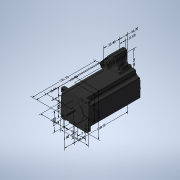
# Autodesk Inventor part: 8156180 EMMT-ST-57-L-RS---(400)
Saved by Autodesk Inventor 2021 (Build 250183000, 183)
## iProperties
Created: 2026-04-24
Part Number: 8156180 EMMT-ST-57-L-RS---(400)
Material: Generic
Catalog Web Link: www.3dfindit.com
Description: EMMT-ST-stepper motor
Vendor: FESTO
Document SubType Name: Modeling
Designer: psAdmin
Manufacturer: FESTO
Mass: 1260 g
Surface Area: 351.744 cm^2
Volume: 333.112 cm^3
Density: 1 g/cm^3
Appearance: PSOLRGB-176-176-176
Category: PARTsolutions
Company: FESTO
Title: 8156180 EMMT-ST-57-L-RS
Author: Cadenas PARTsolutions
Comments: stepper motor
PSOL_IDENT_0: {$CADENAS_DATA/23d-libs/festo/parts/e/emmt/emmt_st.prj},199 {VTYP=3D},{NB=8156180 EMMT-ST-57-L-RS---
PSOL_IDENT_1: (400)},{LINA=8156180 EMMT-ST-57-L-RS},{NN=EMMT-ST},{DATE=09.12.2025 15:36:59},{GEOMDATE=09.12.2025 1
PSOL_IDENT_2: 5:36:20},{VERSION=},{LINEID=200},{WBVAR=LOG},{WBNUMERIC=}  {NB=8156180 EMMT-ST-57-L-RS---(400)},{LIN
PSOL_IDENT_3: A=8156180 EMMT-ST-57-L-RS},{KT=DUMMY},{TNR=8156180},{TYP=EMMT-ST-57-L-RS},{FLA=57},{BAU=L},{ELE=R},{
PSOL_IDENT_4: BRE=-},{LOGDEST=mechanical},{LOG=400},{LOGX='400','High', '300', 'Medium', '200', 'Low'},{B1=56.400}
PSOL_IDENT_5: ,{B2=47.140},{D1=6.350},{D2=38.100},{D3=M17},{D3N=17.000},{D4=5},{D4N=5.000},{H1=88.000},{H3=49.300}
PSOL_IDENT_6: ,{L=131.100},{L1=110.500},{L2=20.600},{L3=1.600},{L4=5.000},{L5=16.700},{L6=33.400},{L7=11.000},{R=3
PSOL_IDENT_7: .000},{L8=0.000},{CNSMASSEXACT=1.260},{GTIN=4052568639686}
NB: 8156180 EMMT-ST-57-L-RS---(400)
NN: EMMT-ST
NT: stepper motor
NBSYN: $TNR. $TYP.---($LOG.)
LINA: 8156180 EMMT-ST-57-L-RS
CATALOG: Festo
TNR: 8156180
TYP: EMMT-ST-57-L-RS
LOG: High
B1: 56.4
B2: 47.14
D1: 6.35
D2: 38.1
D3: M17
D4: 5
H1: 88
H3: 49.3
L: 131.1
L1: 110.5
L2: 20.6
L3: 1.6
L4: 5
L5: 16.7
L6: 33.4
L7: 11
R: 3
CNSMASSEXACT: 1.26
GTIN: 4052568639686
SUPPLIER: FESTO
ARTICLENO: 8156180 EMMT-ST-57-L-RS---(400)
BOMINFO: 8156180 EMMT-ST-57-L-RS
CREATOR: CADENAS GmbH
Autodesk Inventor part; units mm, degrees
sketch "Sketch_1" plane through (0, 0, 0) normal (0, 0, 1) x (1, 0, 0)
  line L0 (-28.2, -28.2) -> (28.2, -28.2)
  line L1 (28.2, -28.2) -> (28.2, 28.2)
  line L2 (28.2, 28.2) -> (-28.2, 28.2)
  line L3 (-28.2, 28.2) -> (-28.2, -28.2)
  constraints: 8 end point
extrude "Extrusion1" add sketch "Sketch_1" against normal blind 110.5
sketch "Sketch_2" plane through (0, 0, -5) normal (0, 0, 1) x (1, 0, 0)
  line L0 (-33.2, -33.2) -> (33.2, -33.2)
  line L1 (33.2, -33.2) -> (33.2, 33.2)
  line L2 (33.2, 33.2) -> (-33.2, 33.2)
  line L3 (-33.2, 33.2) -> (-33.2, -33.2)
  line L4 (-28.2, 19) -> (-28.2, -19)
  line L5 (-28.2, -19) -> (-24, -19)
  arc A0 (-19, -24) -> (-24, -19) centre (-24, -24) ccw
  line L6 (-19, -24) -> (-19, -28.2)
  line L7 (-19, -28.2) -> (19, -28.2)
  line L8 (19, -28.2) -> (19, -24)
  arc A1 (24, -19) -> (19, -24) centre (24, -24) ccw
  line L9 (24, -19) -> (28.2, -19)
  line L10 (28.2, -19) -> (28.2, 19)
  line L11 (28.2, 19) -> (24, 19)
  arc A2 (19, 24) -> (24, 19) centre (24, 24) ccw
  line L12 (19, 24) -> (19, 28.2)
  line L13 (19, 28.2) -> (-19, 28.2)
  line L14 (-19, 28.2) -> (-19, 24)
  arc A3 (-24, 19) -> (-19, 24) centre (-24, 24) ccw
  line L15 (-24, 19) -> (-28.2, 19)
  constraints: 32 end point, 8 point on circle, 4 centre point
extrude "Extrusion2" cut sketch "Sketch_2" against normal blind 105.5
sketch "Sketch_3" plane through (0, 0, -5) normal (0, 0, 1) x (1, 0, 0)
  line L0 (-33.2, -33.2) -> (33.2, -33.2)
  line L1 (33.2, -33.2) -> (33.2, 33.2)
  line L2 (33.2, 33.2) -> (-33.2, 33.2)
  line L3 (-33.2, 33.2) -> (-33.2, -33.2)
  line L4 (-28.2, 16.8) -> (-28.2, -16.8)
  arc A0 (-28.2, -16.8) -> (-26, -19) centre (-26, -16.8) ccw
  line L5 (-26, -19) -> (-24, -19)
  arc A1 (-19, -24) -> (-24, -19) centre (-24, -24) ccw
  line L6 (-19, -24) -> (-19, -26)
  arc A2 (-19, -26) -> (-16.8, -28.2) centre (-16.8, -26) ccw
  line L7 (-16.8, -28.2) -> (16.8, -28.2)
  arc A3 (16.8, -28.2) -> (19, -26) centre (16.8, -26) ccw
  line L8 (19, -26) -> (19, -24)
  arc A4 (24, -19) -> (19, -24) centre (24, -24) ccw
  line L9 (24, -19) -> (26, -19)
  arc A5 (26, -19) -> (28.2, -16.8) centre (26, -16.8) ccw
  line L10 (28.2, -16.8) -> (28.2, 16.8)
  arc A6 (28.2, 16.8) -> (26, 19) centre (26, 16.8) ccw
  line L11 (26, 19) -> (24, 19)
  arc A7 (19, 24) -> (24, 19) centre (24, 24) ccw
  line L12 (19, 24) -> (19, 26)
  arc A8 (19, 26) -> (16.8, 28.2) centre (16.8, 26) ccw
  line L13 (16.8, 28.2) -> (-16.8, 28.2)
  arc A9 (-16.8, 28.2) -> (-19, 26) centre (-16.8, 26) ccw
  line L14 (-19, 26) -> (-19, 24)
  arc A10 (-24, 19) -> (-19, 24) centre (-24, 24) ccw
  line L15 (-24, 19) -> (-26, 19)
  arc A11 (-26, 19) -> (-28.2, 16.8) centre (-26, 16.8) ccw
  constraints: 32 end point, 24 point on circle, 12 centre point
extrude "Extrusion3" cut sketch "Sketch_3" against normal blind 105.5
sketch "Sketch_4" plane through (0, 0, 0) normal (0, 0, 1) x (1, 0, 0)
  line L0 (-33.2, -33.2) -> (33.2, -33.2)
  line L1 (33.2, -33.2) -> (33.2, 33.2)
  line L2 (33.2, 33.2) -> (-33.2, 33.2)
  line L3 (-33.2, 33.2) -> (-33.2, -33.2)
  line L4 (-28.2, 25.2) -> (-28.2, -25.2)
  arc A0 (-28.2, -25.2) -> (-25.2, -28.2) centre (-25.2, -25.2) ccw
  line L5 (-25.2, -28.2) -> (25.2, -28.2)
  arc A1 (25.2, -28.2) -> (28.2, -25.2) centre (25.2, -25.2) ccw
  line L6 (28.2, -25.2) -> (28.2, 25.2)
  arc A2 (28.2, 25.2) -> (25.2, 28.2) centre (25.2, 25.2) ccw
  line L7 (25.2, 28.2) -> (-25.2, 28.2)
  arc A3 (-25.2, 28.2) -> (-28.2, 25.2) centre (-25.2, 25.2) ccw
  constraints: 16 end point, 8 point on circle, 4 centre point
extrude "Extrusion4" cut sketch "Sketch_4" against normal blind 5
sketch "Sketch5" plane through (0, 0, 0) normal (0, 0, 1) x (1, 0, 0)
  point P0 (23.57, 23.57)
hole "Hole1" at (23.57, 23.57, 0) direction (0, 0, -1) diameter 5 depth 5 countersink diameter 6 countersink angle 90
sketch "Sketch6" plane through (0, 0, 0) normal (0, 0, 1) x (1, 0, 0)
  point P0 (23.57, -23.57)
hole "Hole2" at (23.57, -23.57, 0) direction (0, 0, -1) diameter 5 depth 5 countersink diameter 6 countersink angle 90
sketch "Sketch7" plane through (0, 0, 0) normal (0, 0, 1) x (1, 0, 0)
  point P0 (-23.57, 23.57)
hole "Hole3" at (-23.57, 23.57, 0) direction (0, 0, -1) diameter 5 depth 5 countersink diameter 6 countersink angle 90
sketch "Sketch8" plane through (0, 0, 0) normal (0, 0, 1) x (1, 0, 0)
  point P0 (-23.57, -23.57)
hole "Hole4" at (-23.57, -23.57, 0) direction (0, 0, -1) diameter 5 depth 5 countersink diameter 6 countersink angle 90
sketch "Sketch_9" plane through (0, 0, 0) normal (0, 0, 1) x (1, 0, 0)
  arc A0 (12.339, 25.045) -> (18.839, 25.045) centre (15.589, 25.045) ccw
  line L0 (18.839, 25.045) -> (18.839, 28.2)
  line L1 (18.839, 28.2) -> (12.339, 28.2)
  line L2 (12.339, 28.2) -> (12.339, 25.045)
  constraints: 6 end point, 2 point on circle, 1 centre point
extrude "Extrusion5" cut sketch "Sketch_9" against normal blind 2.5
sketch "Sketch_10" plane through (0, 0, 0) normal (0, 0, 1) x (1, 0, 0)
  line L0 (-28.2, 18.839) -> (-28.2, 12.339)
  line L1 (-28.2, 12.339) -> (-25.045, 12.339)
  arc A0 (-25.045, 12.339) -> (-25.045, 18.839) centre (-25.045, 15.589) ccw
  line L2 (-25.045, 18.839) -> (-28.2, 18.839)
  constraints: 6 end point, 2 point on circle, 1 centre point
extrude "Extrusion6" cut sketch "Sketch_10" against normal blind 2.5
sketch "Sketch_11" plane through (0, 0, 0) normal (0, 0, 1) x (1, 0, 0)
  line L0 (-18.839, -25.045) -> (-18.839, -28.2)
  line L1 (-18.839, -28.2) -> (-12.339, -28.2)
  line L2 (-12.339, -28.2) -> (-12.339, -25.045)
  arc A0 (-12.339, -25.045) -> (-18.839, -25.045) centre (-15.589, -25.045) ccw
  constraints: 6 end point, 2 point on circle, 1 centre point
extrude "Extrusion7" cut sketch "Sketch_11" against normal blind 2.5
sketch "Sketch_12" plane through (0, 0, 0) normal (0, 0, 1) x (1, 0, 0)
  arc A0 (25.045, -12.339) -> (25.045, -18.839) centre (25.045, -15.589) ccw
  line L0 (25.045, -18.839) -> (28.2, -18.839)
  line L1 (28.2, -18.839) -> (28.2, -12.339)
  line L2 (28.2, -12.339) -> (25.045, -12.339)
  constraints: 6 end point, 2 point on circle, 1 centre point
extrude "Extrusion8" cut sketch "Sketch_12" against normal blind 2.5
sketch "Sketch_13" plane through (15.589, 0, 0) normal (1, 0, 0) x (0, 0, -1)
  line L0 (2.5, 25.045) -> (0.5, 25.045)
  line L1 (0.5, 25.045) -> (0.5, 27.5284)
  arc A0 (0.5913, 27.628) -> (0.5, 27.5284) centre (0.6, 27.5284) ccw
  line L2 (0.5913, 27.628) -> (2.5, 27.795)
  line L3 (2.5, 27.795) -> (2.5, 25.045)
  line L4 (2.5, 25.045) -> (0.5, 25.045)
  constraints: 10 end point, 2 point on circle, 1 centre point
revolve "Revolution1" add sketch "Sketch_13" angle 360 about axis through (15.589, 25.045, -2.5) along (0, 0, -1)
pattern_linear "Rectangular Pattern1" count 2 spacing 41.7198 along (-0.9739751, -0.2266552, 0) count 2 spacing 41.7198 along (0.2266552, -0.9739751, 0) of "Revolution1"
sketch "Sketch_15" plane through (15.589, 25.045, -0.5) normal (0, 0, 1) x (0, 1, 0)
  line L0 (-2.75, -0.4) -> (2.75, -0.4)
  line L1 (2.75, -0.4) -> (2.75, 0.4)
  line L2 (2.75, 0.4) -> (-2.75, 0.4)
  line L3 (-2.75, 0.4) -> (-2.75, -0.4)
  constraints: 8 end point
extrude "Extrusion9" cut sketch "Sketch_15" against normal blind 0.85
sketch "Pattern_2_SKETCH_1" plane through (-25.045, 15.589, -0.5) normal (0, 0, 1) x (0, 1, 0)
  line L0 (-2.75, -0.4) -> (2.75, -0.4)
  line L1 (2.75, -0.4) -> (2.75, 0.4)
  line L2 (2.75, 0.4) -> (-2.75, 0.4)
  line L3 (-2.75, 0.4) -> (-2.75, -0.4)
  constraints: 8 end point
sketch "Pattern_2_SKETCH_2" plane through (-25.045, 15.589, -0.5) normal (0, 0, 1) x (0, 1, 0)
  line L0 (-43.383, -9.856) -> (-37.883, -9.856)
  line L1 (-37.883, -9.856) -> (-37.883, -9.056)
  line L2 (-37.883, -9.056) -> (-43.383, -9.056)
  line L3 (-43.383, -9.056) -> (-43.383, -9.856)
  constraints: 8 end point
sketch "Pattern_2_SKETCH_3" plane through (-25.045, 15.589, -0.5) normal (0, 0, 1) x (0, 1, 0)
  line L0 (-33.928, -50.49) -> (-28.428, -50.49)
  line L1 (-28.428, -50.49) -> (-28.428, -49.69)
  line L2 (-28.428, -49.69) -> (-33.928, -49.69)
  line L3 (-33.928, -49.69) -> (-33.928, -50.49)
  constraints: 8 end point
extrude "Extrusion10" cut sketch "Pattern_2_SKETCH_1" against normal blind 0.85
extrude "Extrusion11" cut sketch "Pattern_2_SKETCH_2" against normal blind 0.85
extrude "Extrusion12" cut sketch "Pattern_2_SKETCH_3" against normal blind 0.85
sketch "Sketch_17" plane through (0, 0, 0) normal (1, 0, 0) x (0, 1, 0)
  line L0 (0, 0) -> (0, 1.6)
  line L1 (0, 1.6) -> (18.8, 1.6)
  line L2 (18.8, 1.6) -> (19.05, 1.35)
  line L3 (19.05, 1.35) -> (19.05, 0)
  line L4 (19.05, 0) -> (0, 0)
  line L5 (0, 0) -> (0, 1.6)
  constraints: 12 end point
revolve "Revolution2" add sketch "Sketch_17" angle 360 about axis through (0, 0, 0) along (0, 0, -1)
sketch "Sketch19" plane through (0, 0, 1.6) normal (0, 0, 1) x (1, 0, 0)
  point P0 (0, 0)
hole "Hole5" at (0, 0, 1.6) direction (0, 0, -1) diameter 9 depth 5 countersink diameter 10 countersink angle 90
sketch "Sketch_19" plane through (0, 0, 0) normal (1, 0, 0) x (0, 1, 0)
  line L0 (0, -5.4) -> (0, 18.8783)
  line L1 (0, 18.8783) -> (1.25, 19.6)
  line L2 (1.25, 19.6) -> (1.25, 20.6)
  line L3 (1.25, 20.6) -> (2.875, 20.6)
  line L4 (2.875, 20.6) -> (3.175, 20.3)
  line L5 (3.175, 20.3) -> (3.175, -1.4)
  arc A0 (3.175, -1.4) -> (5.175, -3.4) centre (5.175, -1.4) ccw
  line L6 (5.175, -3.4) -> (5.175, -5.4)
  line L7 (5.175, -5.4) -> (0, -5.4)
  line L8 (0, -5.4) -> (0, 18.8783)
  constraints: 18 end point, 2 point on circle, 1 centre point
revolve "Revolution3" add sketch "Sketch_19" angle 360 about axis through (0, 0, -5.4) along (0, 0, -1)
sketch "Sketch_20" plane through (0, 0, 0) normal (1, 0, 0) x (0, 1, 0)
  line L0 (0, -115.5) -> (0, -110.5)
  line L1 (0, -110.5) -> (19.5, -110.5)
  arc A0 (19.5, -110.5) -> (19.9094, -110.287) centre (19.5, -110) ccw
  arc A1 (22.0432, -109.0264) -> (19.9094, -110.287) centre (22.366, -112.009) ccw
  line L2 (22.0432, -109.0264) -> (34.2, -107.8233)
  line L3 (34.2, -107.8233) -> (34.2, -115.5)
  line L4 (34.2, -115.5) -> (0, -115.5)
  line L5 (0, -115.5) -> (0, -110.5)
  constraints: 12 end point, 4 point on circle, 2 centre point
revolve "Revolution4" cut sketch "Sketch_20" angle 360 about axis through (0, 0, -115.5) along (0, 0, -1)
sketch "Sketch_21" plane through (0, 0, -105.2) normal (0, 0, 1) x (1, 0, 0)
  arc A0 (23.4157, 18.3202) -> (27.307, 13.887) centre (24.949, 15.7416) ccw
  arc A1 (28.2, 13.5779) -> (27.307, 13.887) centre (27.7, 13.5779) ccw
  line L0 (28.2, 13.5779) -> (33.2, 13.5779)
  line L1 (33.2, 13.5779) -> (33.2, 25)
  line L2 (33.2, 25) -> (23.1602, 25)
  line L3 (23.1602, 25) -> (23.1602, 19.25)
  arc A2 (23.4157, 18.3202) -> (23.1602, 19.25) centre (23.1602, 18.75) ccw
  constraints: 8 end point, 6 point on circle, 3 centre point
extrude "Extrusion13" cut sketch "Sketch_21" against normal blind 5.3
sketch "Sketch_22" plane through (0, 0, -105.2) normal (0, 0, 1) x (1, 0, 0)
  line L0 (-25, 23.1602) -> (-19.25, 23.1602)
  arc A0 (-18.3202, 23.4157) -> (-19.25, 23.1602) centre (-18.75, 23.1602) ccw
  arc A1 (-18.3202, 23.4157) -> (-13.887, 27.307) centre (-15.7416, 24.949) ccw
  arc A2 (-13.5779, 28.2) -> (-13.887, 27.307) centre (-13.5779, 27.7) ccw
  line L1 (-13.5779, 28.2) -> (-13.5779, 33.2)
  line L2 (-13.5779, 33.2) -> (-25, 33.2)
  line L3 (-25, 33.2) -> (-25, 23.1602)
  constraints: 8 end point, 6 point on circle, 3 centre point
extrude "Extrusion14" cut sketch "Sketch_22" against normal blind 5.3
sketch "Sketch_23" plane through (0, 0, -105.2) normal (0, 0, 1) x (1, 0, 0)
  line L0 (-33.2, -25) -> (-23.1602, -25)
  line L1 (-23.1602, -25) -> (-23.1602, -19.25)
  arc A0 (-23.4157, -18.3202) -> (-23.1602, -19.25) centre (-23.1602, -18.75) ccw
  arc A1 (-23.4157, -18.3202) -> (-27.307, -13.887) centre (-24.949, -15.7416) ccw
  arc A2 (-28.2, -13.5779) -> (-27.307, -13.887) centre (-27.7, -13.5779) ccw
  line L2 (-28.2, -13.5779) -> (-33.2, -13.5779)
  line L3 (-33.2, -13.5779) -> (-33.2, -25)
  constraints: 8 end point, 6 point on circle, 3 centre point
extrude "Extrusion15" cut sketch "Sketch_23" against normal blind 5.3
sketch "Sketch_24" plane through (0, 0, -105.2) normal (0, 0, 1) x (1, 0, 0)
  arc A0 (18.3202, -23.4157) -> (13.887, -27.307) centre (15.7416, -24.949) ccw
  arc A1 (13.5779, -28.2) -> (13.887, -27.307) centre (13.5779, -27.7) ccw
  line L0 (13.5779, -28.2) -> (13.5779, -33.2)
  line L1 (13.5779, -33.2) -> (25, -33.2)
  line L2 (25, -33.2) -> (25, -23.1602)
  line L3 (25, -23.1602) -> (19.25, -23.1602)
  arc A2 (18.3202, -23.4157) -> (19.25, -23.1602) centre (18.75, -23.1602) ccw
  constraints: 8 end point, 6 point on circle, 3 centre point
extrude "Extrusion16" cut sketch "Sketch_24" against normal blind 5.3
sketch "Sketch_25" plane through (0, 0, 0) normal (-0.5336145, 0.8457278, 0) x (0.8457278, 0.5336145, 0)
  line L0 (29.5, 105.2) -> (29.5, 108.2)
  line L1 (29.5, 108.2) -> (31.95, 108.2)
  arc A0 (32.25, 107.9) -> (31.95, 108.2) centre (31.95, 107.9) ccw
  line L2 (32.25, 107.9) -> (32.25, 105.2)
  line L3 (32.25, 105.2) -> (29.5, 105.2)
  line L4 (29.5, 105.2) -> (29.5, 108.2)
  constraints: 10 end point, 2 point on circle, 1 centre point
revolve "Revolution5" add sketch "Sketch_25" angle 360 about axis through (24.949, 15.7416, -105.2) along (0, 0, 1)
pattern_linear "Rectangular Pattern2" count 2 spacing 41.7193 along (-0.9753423, 0.2206974, 0) count 2 spacing 41.7193 along (-0.2206974, -0.9753423, 0) of "Revolution5"
sketch "Sketch_27" plane through (24.949, 15.7416, -108.2) normal (0, 0, -1) x (0.8457278, 0.5336145, 0)
  arc A0 (-1.1621, -0.3564) -> (-0.8897, -0.8282) centre (-0.9699, -0.56) ccw
  arc A1 (-0.2724, -1.1846) -> (-0.8897, -0.8282) centre (-0.7492, -1.2977) ccw
  arc A2 (-0.2724, -1.1846) -> (0.2724, -1.1846) centre (0, -1.12) ccw
  arc A3 (0.8897, -0.8282) -> (0.2724, -1.1846) centre (0.7492, -1.2977) ccw
  arc A4 (0.8897, -0.8282) -> (1.1621, -0.3564) centre (0.9699, -0.56) ccw
  arc A5 (1.1621, 0.3564) -> (1.1621, -0.3564) centre (1.4984, 0) ccw
  arc A6 (1.1621, 0.3564) -> (0.8897, 0.8282) centre (0.9699, 0.56) ccw
  arc A7 (0.2724, 1.1846) -> (0.8897, 0.8282) centre (0.7492, 1.2977) ccw
  arc A8 (0.2724, 1.1846) -> (-0.2724, 1.1846) centre (0, 1.12) ccw
  arc A9 (-0.8897, 0.8282) -> (-0.2724, 1.1846) centre (-0.7492, 1.2977) ccw
  arc A10 (-0.8897, 0.8282) -> (-1.1621, 0.3564) centre (-0.9699, 0.56) ccw
  arc A11 (-1.1621, -0.3564) -> (-1.1621, 0.3564) centre (-1.4984, 0) ccw
  constraints: 24 point on circle, 12 centre point
extrude "Extrusion17" cut sketch "Sketch_27" against normal blind 1.65
pattern_linear "Rectangular Pattern3" count 2 spacing 41.7193 along (-0.2206974, -0.9753423, 0) count 2 spacing 41.7193 along (-0.9753423, 0.2206974, 0) of "Extrusion17"
sketch "Sketch_29" plane through (0, 28.2, 0) normal (0, 1, 0) x (1, 0, 0)
  arc A0 (-13, 82.8) -> (-11, 80.8) centre (-11, 82.8) ccw
  line L0 (-11, 80.8) -> (11, 80.8)
  arc A1 (11, 80.8) -> (13, 82.8) centre (11, 82.8) ccw
  line L1 (13, 82.8) -> (13, 104.8)
  arc A2 (13, 104.8) -> (11, 106.8) centre (11, 104.8) ccw
  line L2 (11, 106.8) -> (-11, 106.8)
  arc A3 (-11, 106.8) -> (-13, 104.8) centre (-11, 104.8) ccw
  line L3 (-13, 104.8) -> (-13, 82.8)
  constraints: 8 end point, 8 point on circle, 4 centre point
extrude "Extrusion18" add sketch "Sketch_29" along normal blind 1.2
sketch "Sketch_30" plane through (0, 28.2, 0) normal (0, 1, 0) x (1, 0, 0)
  arc A0 (-12.85, 82.95) -> (-10.85, 80.95) centre (-10.85, 82.95) ccw
  line L0 (-10.85, 80.95) -> (10.85, 80.95)
  arc A1 (10.85, 80.95) -> (12.85, 82.95) centre (10.85, 82.95) ccw
  line L1 (12.85, 82.95) -> (12.85, 104.65)
  arc A2 (12.85, 104.65) -> (10.85, 106.65) centre (10.85, 104.65) ccw
  line L2 (10.85, 106.65) -> (-10.85, 106.65)
  arc A3 (-10.85, 106.65) -> (-12.85, 104.65) centre (-10.85, 104.65) ccw
  line L3 (-12.85, 104.65) -> (-12.85, 82.95)
  constraints: 8 end point, 8 point on circle, 4 centre point
extrude "Extrusion19" add sketch "Sketch_30" along normal blind 9.6
sketch "Sketch_31" plane through (0, 0, 0) normal (1, 0, 0) x (0, 1, 0)
  line L0 (39.8, -93.8) -> (37.8, -93.8)
  line L1 (37.8, -93.8) -> (37.8, -82.7)
  line L2 (37.8, -82.7) -> (31.9, -79.6769)
  line L3 (31.9, -79.6769) -> (31.9, -73.8)
  line L4 (31.9, -73.8) -> (39.8, -73.8)
  line L5 (39.8, -73.8) -> (39.8, -93.8)
  line L6 (39.8, -93.8) -> (37.8, -93.8)
  constraints: 14 end point
revolve "Revolution6" cut sketch "Sketch_31" angle 360 about axis through (0, 39.8, -93.8) along (0, 1, 0)
sketch "Sketch_32" plane through (0, 0, 0) normal (1, 0, 0) x (0, 1, 0)
  line L0 (40.8, -78.8) -> (31.9, -78.8)
  line L1 (31.9, -78.8) -> (31.9, -80.95)
  line L2 (31.9, -80.95) -> (37.8, -81.7792)
  line L3 (37.8, -81.7792) -> (37.8, -105.8208)
  line L4 (37.8, -105.8208) -> (31.9, -106.65)
  line L5 (31.9, -106.65) -> (31.9, -108.8)
  line L6 (31.9, -108.8) -> (40.8, -108.8)
  line L7 (40.8, -108.8) -> (40.8, -78.8)
  constraints: 16 end point
extrude "Extrusion20" cut sketch "Sketch_32" along normal mid plane 11.4
sketch "Sketch_33" plane through (0, 0, -93.8) normal (0, 0, 1) x (1, 0, 0)
  line L0 (-15, 40.8) -> (-15, 31.9)
  line L1 (-15, 31.9) -> (-12.85, 31.9)
  line L2 (-12.85, 31.9) -> (-12.0208, 37.8)
  line L3 (-12.0208, 37.8) -> (12.0208, 37.8)
  line L4 (12.0208, 37.8) -> (12.85, 31.9)
  line L5 (12.85, 31.9) -> (15, 31.9)
  line L6 (15, 31.9) -> (15, 40.8)
  line L7 (15, 40.8) -> (-15, 40.8)
  constraints: 16 end point
extrude "Extrusion21" cut sketch "Sketch_33" along normal mid plane 11.4
sketch "Sketch_34" plane through (0, 31.9, 0) normal (0, 1, 0) x (1, 0, 0)
  line L0 (-14.6995, 108.4995) -> (-14.6995, 79.1005)
  line L1 (-14.6995, 79.1005) -> (14.6995, 79.1005)
  line L2 (14.6995, 79.1005) -> (14.6995, 108.4995)
  line L3 (14.6995, 108.4995) -> (-14.6995, 108.4995)
  line L4 (-13.6995, 100.4995) -> (-13.6995, 87.1005)
  line L5 (-13.6995, 87.1005) -> (-9.8995, 87.1005)
  arc A0 (-6.6995, 83.9005) -> (-9.8995, 87.1005) centre (-9.8995, 83.9005) ccw
  line L6 (-6.6995, 83.9005) -> (-6.6995, 80.1005)
  line L7 (-6.6995, 80.1005) -> (6.6995, 80.1005)
  line L8 (6.6995, 80.1005) -> (6.6995, 83.9005)
  arc A1 (9.8995, 87.1005) -> (6.6995, 83.9005) centre (9.8995, 83.9005) ccw
  line L9 (9.8995, 87.1005) -> (13.6995, 87.1005)
  line L10 (13.6995, 87.1005) -> (13.6995, 100.4995)
  line L11 (13.6995, 100.4995) -> (9.8995, 100.4995)
  arc A2 (6.6995, 103.6995) -> (9.8995, 100.4995) centre (9.8995, 103.6995) ccw
  line L12 (6.6995, 103.6995) -> (6.6995, 107.4995)
  line L13 (6.6995, 107.4995) -> (-6.6995, 107.4995)
  line L14 (-6.6995, 107.4995) -> (-6.6995, 103.6995)
  arc A3 (-9.8995, 100.4995) -> (-6.6995, 103.6995) centre (-9.8995, 103.6995) ccw
  line L15 (-9.8995, 100.4995) -> (-13.6995, 100.4995)
  constraints: 32 end point, 8 point on circle, 4 centre point
extrude "Extrusion22" cut sketch "Sketch_34" along normal blind 5.7
sketch "Sketch_35" plane through (9.9, 0, 0) normal (1, 0, 0) x (0, 0, -1)
  line L0 (83.9, 31.9) -> (83.9, 34.3)
  line L1 (83.9, 34.3) -> (85.4, 34.3)
  arc A0 (86.8675, 33.7304) -> (85.4, 34.3) centre (85.4, 32.125) ccw
  arc A1 (86.9, 33.6565) -> (86.8675, 33.7304) centre (86.8, 33.6565) ccw
  line L2 (86.9, 33.6565) -> (86.9, 31.9)
  line L3 (86.9, 31.9) -> (83.9, 31.9)
  line L4 (83.9, 31.9) -> (83.9, 34.3)
  constraints: 10 end point, 4 point on circle, 2 centre point
revolve "Revolution7" add sketch "Sketch_35" angle 360 about axis through (9.9, 31.9, -83.9) along (0, -1, 0)
sketch "Pattern_5_SKETCH_1" plane through (9.8995, 0, -19.7995) normal (1, 0, 0) x (0, 0, -1)
  line L0 (83.9, 31.9) -> (83.9, 34.3)
  line L1 (83.9, 34.3) -> (85.4, 34.3)
  arc A0 (86.8675, 33.7304) -> (85.4, 34.3) centre (85.4, 32.125) ccw
  arc A1 (86.9, 33.6565) -> (86.8675, 33.7304) centre (86.8, 33.6565) ccw
  line L2 (86.9, 33.6565) -> (86.9, 31.9)
  line L3 (86.9, 31.9) -> (83.9, 31.9)
  line L4 (83.9, 31.9) -> (83.9, 34.3)
  constraints: 10 end point, 4 point on circle, 2 centre point
sketch "Pattern_5_SKETCH_2" plane through (-9.8995, 0, -19.7995) normal (1, 0, 0) x (0, 0, -1)
  line L0 (83.9, 31.9) -> (83.9, 34.3)
  line L1 (83.9, 34.3) -> (85.4, 34.3)
  arc A0 (86.8675, 33.7304) -> (85.4, 34.3) centre (85.4, 32.125) ccw
  arc A1 (86.9, 33.6565) -> (86.8675, 33.7304) centre (86.8, 33.6565) ccw
  line L2 (86.9, 33.6565) -> (86.9, 31.9)
  line L3 (86.9, 31.9) -> (83.9, 31.9)
  line L4 (83.9, 31.9) -> (83.9, 34.3)
  constraints: 10 end point, 4 point on circle, 2 centre point
sketch "Pattern_5_SKETCH_3" plane through (-9.8995, 0, -19.7995) normal (1, 0, 0) x (0, 0, -1)
  line L0 (64.101, 31.9) -> (64.101, 34.3)
  line L1 (64.101, 34.3) -> (65.601, 34.3)
  arc A0 (67.0685, 33.7304) -> (65.601, 34.3) centre (65.601, 32.125) ccw
  arc A1 (67.101, 33.6565) -> (67.0685, 33.7304) centre (67.001, 33.6565) ccw
  line L2 (67.101, 33.6565) -> (67.101, 31.9)
  line L3 (67.101, 31.9) -> (64.101, 31.9)
  line L4 (64.101, 31.9) -> (64.101, 34.3)
  constraints: 10 end point, 4 point on circle, 2 centre point
revolve "Revolution8" add sketch "Pattern_5_SKETCH_1" angle 360 about axis through (9.8995, 31.9, -103.6995) along (0, -1, 0)
revolve "Revolution9" add sketch "Pattern_5_SKETCH_2" angle 360 about axis through (-9.8995, 31.9, -103.6995) along (0, -1, 0)
revolve "Revolution10" add sketch "Pattern_5_SKETCH_3" angle 360 about axis through (-9.8995, 31.9, -83.9005) along (0, -1, 0)
sketch "Sketch_37" plane through (9.9, 34.3, -83.9) normal (0, 1, 0) x (0, 0, -1)
  arc A0 (-1.1621, -0.3564) -> (-0.8897, -0.8282) centre (-0.9699, -0.56) ccw
  arc A1 (-0.2724, -1.1846) -> (-0.8897, -0.8282) centre (-0.7492, -1.2977) ccw
  arc A2 (-0.2724, -1.1846) -> (0.2724, -1.1846) centre (0, -1.12) ccw
  arc A3 (0.8897, -0.8282) -> (0.2724, -1.1846) centre (0.7492, -1.2977) ccw
  arc A4 (0.8897, -0.8282) -> (1.1621, -0.3564) centre (0.9699, -0.56) ccw
  arc A5 (1.1621, 0.3564) -> (1.1621, -0.3564) centre (1.4984, 0) ccw
  arc A6 (1.1621, 0.3564) -> (0.8897, 0.8282) centre (0.9699, 0.56) ccw
  arc A7 (0.2724, 1.1846) -> (0.8897, 0.8282) centre (0.7492, 1.2977) ccw
  arc A8 (0.2724, 1.1846) -> (-0.2724, 1.1846) centre (0, 1.12) ccw
  arc A9 (-0.8897, 0.8282) -> (-0.2724, 1.1846) centre (-0.7492, 1.2977) ccw
  arc A10 (-0.8897, 0.8282) -> (-1.1621, 0.3564) centre (-0.9699, 0.56) ccw
  arc A11 (-1.1621, -0.3564) -> (-1.1621, 0.3564) centre (-1.4984, 0) ccw
  constraints: 24 point on circle, 12 centre point
extrude "Extrusion23" cut sketch "Sketch_37" against normal blind 1.65
pattern_linear "Rectangular Pattern4" count 2 spacing 19.799 along (0, 0, -1) count 2 spacing 19.799 along (-1, 0, 0) of "Extrusion23"
sketch "Sketch_39" plane through (9.9, 34.3, -83.9) normal (0, 1, 0) x (0, 0, -1)
  line L0 (-2.3925, -0.5) -> (2.3925, -0.5)
  line L1 (2.3925, -0.5) -> (2.3925, 0.5)
  line L2 (2.3925, 0.5) -> (-2.3925, 0.5)
  line L3 (-2.3925, 0.5) -> (-2.3925, -0.5)
  constraints: 8 end point
extrude "Extrusion24" cut sketch "Sketch_39" against normal blind 1
pattern_linear "Rectangular Pattern5" count 2 spacing 19.799 along (0, 0, -1) count 2 spacing 19.799 along (-1, 0, 0) of "Extrusion24"
sketch "Sketch_41" plane through (0, 0, 0) normal (1, 0, 0) x (0, 1, 0)
  line L0 (37.8, -93.8) -> (49.3, -93.8)
  line L1 (49.3, -93.8) -> (49.3, -103.6)
  line L2 (49.3, -103.6) -> (39.3, -103.6)
  line L3 (39.3, -103.6) -> (39.3, -104.15)
  line L4 (39.3, -104.15) -> (37.8, -104.15)
  line L5 (37.8, -104.15) -> (37.8, -93.8)
  line L6 (37.8, -93.8) -> (49.3, -93.8)
  constraints: 14 end point
revolve "Revolution11" add sketch "Sketch_41" angle 360 about axis through (0, 37.8, -93.8) along (0, -1, 0)
sketch "Sketch_42" plane through (0, 0, -104.8) normal (0, 0, 1) x (1, 0, 0)
  arc A0 (-5.5338, 57.4486) -> (-2.9432, 39.9) centre (0, 49.3) ccw
  line L0 (-2.9432, 39.9) -> (2.9432, 39.9)
  arc A1 (2.9432, 39.9) -> (5.5338, 57.4486) centre (0, 49.3) ccw
  arc A2 (4.0145, 59.3672) -> (5.5338, 57.4486) centre (8.3, 61.2) ccw
  arc A3 (4.0145, 59.3672) -> (-4.0145, 59.3672) centre (0, 40.965) ccw
  arc A4 (-5.5338, 57.4486) -> (-4.0145, 59.3672) centre (-8.3, 61.2) ccw
  constraints: 10 point on circle, 5 centre point, 2 end point
extrude "Extrusion25" add sketch "Sketch_42" along normal blind 28.5
sketch "Sketch_43" plane through (0, 39.3, 0) normal (0, 1, 0) x (1, 0, 0)
  line L0 (-12, 94.75) -> (-9.9999, 94.75)
  arc A0 (9.9999, 94.75) -> (-9.9999, 94.75) centre (0, 94.8) ccw
  line L1 (9.9999, 94.75) -> (12, 94.75)
  line L2 (12, 94.75) -> (12, 110.5)
  line L3 (12, 110.5) -> (-12, 110.5)
  line L4 (-12, 110.5) -> (-12, 94.75)
  constraints: 10 end point, 2 point on circle, 1 centre point
extrude "Extrusion26" cut sketch "Sketch_43" along normal blind 21
sketch "Sketch_44" plane through (0, 0, 0) normal (1, 0, 0) x (0, 1, 0)
  line L0 (49.3, -76.3) -> (49.3, -62.94)
  line L1 (49.3, -62.94) -> (56.175, -62.94)
  line L2 (56.175, -62.94) -> (56.175, -60.6)
  line L3 (56.175, -60.6) -> (56.375, -60.4)
  line L4 (56.375, -60.4) -> (57.07, -60.4)
  line L5 (57.07, -60.4) -> (57.07, -70.0237)
  arc A0 (57.07, -70.0237) -> (57.1303, -70.3657) centre (58.07, -70.0237) ccw
  line L6 (57.1303, -70.3657) -> (57.2397, -70.6662)
  arc A1 (57.3, -71.0082) -> (57.2397, -70.6662) centre (56.3, -71.0082) ccw
  line L7 (57.3, -71.0082) -> (57.3, -76.3)
  line L8 (57.3, -76.3) -> (49.3, -76.3)
  line L9 (49.3, -76.3) -> (49.3, -62.94)
  constraints: 20 end point, 4 point on circle, 2 centre point
revolve "Revolution12" add sketch "Sketch_44" angle 360 about axis through (0, 49.3, -76.3) along (0, 0, -1)
sketch "Sketch_45" plane through (0, 0, 0) normal (1, 0, 0) x (0, 1, 0)
  line L0 (49.3, -74.1) -> (49.3, -64.3)
  line L1 (49.3, -64.3) -> (57.1865, -64.3)
  line L2 (57.1865, -64.3) -> (57.8, -64.9135)
  line L3 (57.8, -64.9135) -> (57.8, -70.3)
  line L4 (57.8, -70.3) -> (58.3, -70.3)
  line L5 (58.3, -70.3) -> (58.3, -70.8)
  line L6 (58.3, -70.8) -> (57.4, -70.8)
  line L7 (57.4, -70.8) -> (57.4, -72.4)
  line L8 (57.4, -72.4) -> (58.3, -72.4)
  line L9 (58.3, -72.4) -> (58.3, -74.1)
  line L10 (58.3, -74.1) -> (49.3, -74.1)
  line L11 (49.3, -74.1) -> (49.3, -64.3)
  constraints: 24 end point
revolve "Revolution13" add sketch "Sketch_45" angle 190 about axis through (0, 49.3, -74.1) along (0, 0, 1)
thread "Thread1" size "M17x1" class "6g" standard "ISO Metric profile" full length
sketch "Sketch_46" plane through (0, 49.3, 0) normal (-0.889097, 0.4577187, 0) x (0.4577187, 0.889097, 0)
  line L0 (0, 64.3) -> (0, 74.1)
  line L1 (0, 74.1) -> (9, 74.1)
  line L2 (9, 74.1) -> (9, 72.4)
  line L3 (9, 72.4) -> (8.1, 72.4)
  line L4 (8.1, 72.4) -> (8.1, 70.8)
  line L5 (8.1, 70.8) -> (9, 70.8)
  line L6 (9, 70.8) -> (9, 70.3)
  line L7 (9, 70.3) -> (8.5, 70.3)
  line L8 (8.5, 70.3) -> (8.5, 64.9135)
  line L9 (8.5, 64.9135) -> (7.8865, 64.3)
  line L10 (7.8865, 64.3) -> (0, 64.3)
  line L11 (0, 64.3) -> (0, 74.1)
  constraints: 24 end point
revolve "Revolution14" add sketch "Sketch_46" angle 116.5 about axis through (0, 49.3, -64.3) along (0, 0, -1)
thread "Thread2" size "M17x1" class "6g" standard "ISO Metric profile" full length
sketch "Sketch_47" plane through (0, 49.3, -62.94) normal (0, 0, 1) x (0, 1, 0)
  line L0 (-6.1, 1) -> (-6.1, -1)
  arc A0 (-6.1, -1) -> (-5.399, -2.3755) centre (-4.4, -1) ccw
  arc A1 (-5.201, -2.8701) -> (-5.399, -2.3755) centre (-5.6929, -2.78) ccw
  arc A2 (-5.201, -2.8701) -> (-4.7227, -4.4661) centre (-3.4, -3.2) ccw
  arc A3 (-4.7227, -4.4661) -> (0.9057, -6.4366) centre (0, 0) ccw
  arc A4 (0.9057, -6.4366) -> (1.25, -6.0405) centre (0.85, -6.0405) ccw
  line L1 (1.25, -6.0405) -> (1.25, -4.4533)
  arc A5 (1.8271, -1.8515) -> (1.25, -4.4533) centre (3.25, -3.532) ccw
  arc A6 (1.8271, -1.8515) -> (1.8271, 1.8515) centre (0.3, 0) ccw
  arc A7 (1.25, 4.4533) -> (1.8271, 1.8515) centre (3.25, 3.532) ccw
  line L2 (1.25, 4.4533) -> (1.25, 6.0405)
  arc A8 (1.25, 6.0405) -> (0.9057, 6.4366) centre (0.85, 6.0405) ccw
  arc A9 (0.9057, 6.4366) -> (-4.7227, 4.4661) centre (0, 0) ccw
  arc A10 (-4.7227, 4.4661) -> (-5.201, 2.8701) centre (-3.4, 3.2) ccw
  arc A11 (-5.399, 2.3755) -> (-5.201, 2.8701) centre (-5.6929, 2.78) ccw
  arc A12 (-5.399, 2.3755) -> (-6.1, 1) centre (-4.4, 1) ccw
  constraints: 26 point on circle, 13 centre point, 6 end point
extrude "Extrusion27" cut sketch "Sketch_47" against normal blind 2.05
sketch "Sketch_48" plane through (0, 49.3, -62.94) normal (0, 0, 1) x (0, 1, 0)
  arc A0 (-2.325, -2.248) -> (-4.3467, -4.2798) centre (-3.4, -3.2) ccw
  arc A1 (-4.3467, -4.2798) -> (-1.0444, -6.0099) centre (0, 0) ccw
  arc A2 (-1.0444, -6.0099) -> (-0.9228, -3.0666) centre (-0.7, -4.55) ccw
  arc A3 (-1.0662, -3.0532) -> (-0.9228, -3.0666) centre (-0.9673, -2.77) ccw
  arc A4 (-2.325, -2.248) -> (-1.0662, -3.0532) centre (0, 0) ccw
  constraints: 10 point on circle, 5 centre point
extrude "Extrusion28" cut sketch "Sketch_48" against normal blind 5.6
sketch "Sketch_49" plane through (0, 49.3, -62.94) normal (0, 0, 1) x (0, 1, 0)
  arc A0 (-4.3467, 4.2798) -> (-2.325, 2.248) centre (-3.4, 3.2) ccw
  arc A1 (-1.0662, 3.0532) -> (-2.325, 2.248) centre (0, 0) ccw
  arc A2 (-0.9228, 3.0666) -> (-1.0662, 3.0532) centre (-0.9673, 2.77) ccw
  arc A3 (-0.9228, 3.0666) -> (-1.0444, 6.0099) centre (-0.7, 4.55) ccw
  arc A4 (-1.0444, 6.0099) -> (-4.3467, 4.2798) centre (0, 0) ccw
  constraints: 10 point on circle, 5 centre point
extrude "Extrusion29" cut sketch "Sketch_49" against normal blind 5.6
sketch "Sketch_50" plane through (0, 49.3, -62.94) normal (0, 0, 1) x (0, 1, 0)
  line L0 (-5.5, 1) -> (-5.5, -1)
  arc A0 (-5.5, -1) -> (-4.8497, -2.0039) centre (-4.4, -1) ccw
  arc A1 (-4.7488, -2.105) -> (-4.8497, -2.0039) centre (-4.9315, -2.1864) ccw
  line L1 (-4.7488, -2.105) -> (-4.3503, -3)
  line L2 (-4.3503, -3) -> (-2.4566, -3)
  line L3 (-2.4566, -3) -> (-0.356, 0)
  line L4 (-0.356, 0) -> (-2.4566, 3)
  line L5 (-2.4566, 3) -> (-4.3503, 3)
  line L6 (-4.3503, 3) -> (-4.7488, 2.105)
  arc A2 (-4.8497, 2.0039) -> (-4.7488, 2.105) centre (-4.9315, 2.1864) ccw
  arc A3 (-4.8497, 2.0039) -> (-5.5, 1) centre (-4.4, 1) ccw
  constraints: 14 end point, 8 point on circle, 4 centre point
extrude "Extrusion30" cut sketch "Sketch_50" against normal blind 3.5
sketch "Sketch_51" plane through (0, 0, 0) normal (1, 0, 0) x (0, 1, 0)
  line L0 (49.6, -68.04) -> (49.6, -64.99)
  line L1 (49.6, -64.99) -> (51.4, -64.99)
  arc A0 (51.4, -64.99) -> (51.25, -65.14) centre (51.4, -65.14) ccw
  line L2 (51.25, -65.14) -> (51.25, -67.84)
  arc A1 (51.05, -68.04) -> (51.25, -67.84) centre (51.05, -67.84) ccw
  line L3 (51.05, -68.04) -> (49.6, -68.04)
  line L4 (49.6, -68.04) -> (49.6, -64.99)
  constraints: 10 end point, 4 point on circle, 2 centre point
revolve "Revolution15" cut sketch "Sketch_51" angle 360 about axis through (0, 49.6, -68.04) along (0, 0, -1)
sketch "Sketch_52" plane through (0, 49.3, -62.94) normal (0, 0, 1) x (0, 1, 0)
  arc A0 (4.1103, 1.4714) -> (4.1103, -1.4714) centre (4.8, 0) ccw
  arc A1 (5.3016, -2.6503) -> (4.1103, -1.4714) centre (3.25, -3.532) ccw
  arc A2 (5.3016, -2.6503) -> (5.8504, -2.6559) centre (5.5772, -2.5319) ccw
  arc A3 (5.8504, -2.6559) -> (5.8504, 2.6559) centre (0, 0) ccw
  arc A4 (5.8504, 2.6559) -> (5.3016, 2.6503) centre (5.5772, 2.5319) ccw
  arc A5 (4.1103, 1.4714) -> (5.3016, 2.6503) centre (3.25, 3.532) ccw
  constraints: 12 point on circle, 6 centre point
extrude "Extrusion31" cut sketch "Sketch_52" against normal blind 5.6
sketch "Sketch_53" plane through (0, 52.55, 0) normal (0, 1, 0) x (1, 0, 0)
  line L0 (3.532, 62.94) -> (3.532, 68.54)
  line L1 (3.532, 68.54) -> (5.157, 68.54)
  line L2 (5.157, 68.54) -> (5.157, 63.14)
  arc A0 (5.157, 63.14) -> (5.357, 62.94) centre (5.357, 63.14) ccw
  line L3 (5.357, 62.94) -> (3.532, 62.94)
  line L4 (3.532, 62.94) -> (3.532, 68.54)
  constraints: 10 end point, 2 point on circle, 1 centre point
revolve "Revolution16" cut sketch "Sketch_53" angle 360 about axis through (3.532, 52.55, -62.94) along (0, 0, 1)
sketch "Sketch_54" plane through (0, 52.55, 0) normal (0, 1, 0) x (1, 0, 0)
  line L0 (-3.532, 62.94) -> (-3.532, 68.54)
  line L1 (-3.532, 68.54) -> (-1.907, 68.54)
  line L2 (-1.907, 68.54) -> (-1.907, 63.14)
  arc A0 (-1.907, 63.14) -> (-1.707, 62.94) centre (-1.707, 63.14) ccw
  line L3 (-1.707, 62.94) -> (-3.532, 62.94)
  line L4 (-3.532, 62.94) -> (-3.532, 68.54)
  constraints: 10 end point, 2 point on circle, 1 centre point
revolve "Revolution17" cut sketch "Sketch_54" angle 360 about axis through (-3.532, 52.55, -62.94) along (0, 0, 1)
sketch "Sketch_55" plane through (0, 0, 0) normal (1, 0, 0) x (0, 1, 0)
  line L0 (49.6, -68.04) -> (49.6, -63.36)
  line L1 (49.6, -63.36) -> (49.85, -63.36)
  arc A0 (50.1, -64.06) -> (49.85, -63.36) centre (49.1007, -64.0222) ccw
  line L2 (50.1, -64.06) -> (50.1, -68.04)
  line L3 (50.1, -68.04) -> (49.6, -68.04)
  line L4 (49.6, -68.04) -> (49.6, -63.36)
  constraints: 10 end point, 2 point on circle, 1 centre point
revolve "Revolution18" add sketch "Sketch_55" angle 360 about axis through (0, 49.6, -68.04) along (0, 0, -1)
sketch "Pattern_8_SKETCH_1" plane through (0, 4.5, -0.5) normal (1, 0, 0) x (0, 0, -1)
  line L0 (68.04, 49.6) -> (63.36, 49.6)
  line L1 (63.36, 49.6) -> (63.36, 49.85)
  arc A0 (64.06, 50.1) -> (63.36, 49.85) centre (64.0222, 49.1007) ccw
  line L2 (64.06, 50.1) -> (68.04, 50.1)
  line L3 (68.04, 50.1) -> (68.04, 49.6)
  line L4 (68.04, 49.6) -> (63.36, 49.6)
  constraints: 10 end point, 2 point on circle, 1 centre point
sketch "Pattern_8_SKETCH_2" plane through (3.532, 2.95, -0.5) normal (1, 0, 0) x (0, 0, -1)
  line L0 (68.04, 49.6) -> (63.36, 49.6)
  line L1 (63.36, 49.6) -> (63.36, 49.85)
  arc A0 (64.06, 50.1) -> (63.36, 49.85) centre (64.0222, 49.1007) ccw
  line L2 (64.06, 50.1) -> (68.04, 50.1)
  line L3 (68.04, 50.1) -> (68.04, 49.6)
  line L4 (68.04, 49.6) -> (63.36, 49.6)
  constraints: 10 end point, 2 point on circle, 1 centre point
sketch "Pattern_8_SKETCH_3" plane through (-3.532, 2.95, -0.5) normal (1, 0, 0) x (0, 0, -1)
  line L0 (68.04, 49.6) -> (63.36, 49.6)
  line L1 (63.36, 49.6) -> (63.36, 49.85)
  arc A0 (64.06, 50.1) -> (63.36, 49.85) centre (64.0222, 49.1007) ccw
  line L2 (64.06, 50.1) -> (68.04, 50.1)
  line L3 (68.04, 50.1) -> (68.04, 49.6)
  line L4 (68.04, 49.6) -> (63.36, 49.6)
  constraints: 10 end point, 2 point on circle, 1 centre point
sketch "Pattern_8_SKETCH_4" plane through (-4.55, -1, -0.5) normal (1, 0, 0) x (0, 0, -1)
  line L0 (68.04, 49.6) -> (63.36, 49.6)
  line L1 (63.36, 49.6) -> (63.36, 49.85)
  arc A0 (64.06, 50.1) -> (63.36, 49.85) centre (64.0222, 49.1007) ccw
  line L2 (64.06, 50.1) -> (68.04, 50.1)
  line L3 (68.04, 50.1) -> (68.04, 49.6)
  line L4 (68.04, 49.6) -> (63.36, 49.6)
  constraints: 10 end point, 2 point on circle, 1 centre point
sketch "Pattern_8_SKETCH_5" plane through (4.55, -1, -0.5) normal (1, 0, 0) x (0, 0, -1)
  line L0 (68.04, 49.6) -> (63.36, 49.6)
  line L1 (63.36, 49.6) -> (63.36, 49.85)
  arc A0 (64.06, 50.1) -> (63.36, 49.85) centre (64.0222, 49.1007) ccw
  line L2 (64.06, 50.1) -> (68.04, 50.1)
  line L3 (68.04, 50.1) -> (68.04, 49.6)
  line L4 (68.04, 49.6) -> (63.36, 49.6)
  constraints: 10 end point, 2 point on circle, 1 centre point
sketch "Pattern_8_SKETCH_6" plane through (-3.2, -3.7, -0.5) normal (1, 0, 0) x (0, 0, -1)
  line L0 (68.04, 49.6) -> (63.36, 49.6)
  line L1 (63.36, 49.6) -> (63.36, 49.85)
  arc A0 (64.06, 50.1) -> (63.36, 49.85) centre (64.0222, 49.1007) ccw
  line L2 (64.06, 50.1) -> (68.04, 50.1)
  line L3 (68.04, 50.1) -> (68.04, 49.6)
  line L4 (68.04, 49.6) -> (63.36, 49.6)
  constraints: 10 end point, 2 point on circle, 1 centre point
sketch "Pattern_8_SKETCH_7" plane through (3.2, -3.7, -0.5) normal (1, 0, 0) x (0, 0, -1)
  line L0 (68.04, 49.6) -> (63.36, 49.6)
  line L1 (63.36, 49.6) -> (63.36, 49.85)
  arc A0 (64.06, 50.1) -> (63.36, 49.85) centre (64.0222, 49.1007) ccw
  line L2 (64.06, 50.1) -> (68.04, 50.1)
  line L3 (68.04, 50.1) -> (68.04, 49.6)
  line L4 (68.04, 49.6) -> (63.36, 49.6)
  constraints: 10 end point, 2 point on circle, 1 centre point
revolve "Revolution19" add sketch "Pattern_8_SKETCH_1" angle 360 about axis through (0, 54.1, -68.54) along (0, 0, -1)
revolve "Revolution20" add sketch "Pattern_8_SKETCH_2" angle 360 about axis through (3.532, 52.55, -68.54) along (0, 0, -1)
revolve "Revolution21" add sketch "Pattern_8_SKETCH_3" angle 360 about axis through (-3.532, 52.55, -68.54) along (0, 0, -1)
revolve "Revolution22" add sketch "Pattern_8_SKETCH_4" angle 360 about axis through (-4.55, 48.6, -68.54) along (0, 0, -1)
revolve "Revolution23" add sketch "Pattern_8_SKETCH_5" angle 360 about axis through (4.55, 48.6, -68.54) along (0, 0, -1)
revolve "Revolution24" add sketch "Pattern_8_SKETCH_6" angle 360 about axis through (-3.2, 45.9, -68.54) along (0, 0, -1)
revolve "Revolution25" add sketch "Pattern_8_SKETCH_7" angle 360 about axis through (3.2, 45.9, -68.54) along (0, 0, -1)
sketch "Sketch_57" plane through (1, 0, 0) normal (1, 0, 0) x (0, 0, -1)
  line L0 (66.44, 44.9) -> (63.19, 44.9)
  line L1 (63.19, 44.9) -> (63.19, 45)
  arc A0 (63.59, 45.2) -> (63.19, 45) centre (63.59, 44.7) ccw
  line L2 (63.59, 45.2) -> (66.44, 45.2)
  line L3 (66.44, 45.2) -> (66.44, 44.9)
  line L4 (66.44, 44.9) -> (63.19, 44.9)
  constraints: 10 end point, 2 point on circle, 1 centre point
revolve "Revolution26" add sketch "Sketch_57" angle 360 about axis through (1, 44.9, -66.44) along (0, 0, -1)
pattern_linear "Rectangular Pattern6" count 2 spacing 2 along (0, 1, 0) count 2 spacing 2 along (-1, 0, 0) of "Revolution26"
sketch "Sketch_59" plane through (0, 0, -64.3) normal (0, 0, 1) x (1, 0, 0)
  line L0 (7.4404, 44.3) -> (10.79, 44.3)
  line L1 (10.79, 44.3) -> (10.79, 54.3)
  line L2 (10.79, 54.3) -> (7.4404, 54.3)
  line L3 (7.4404, 54.3) -> (7.7694, 49.5941)
  arc A0 (7.7694, 49.0059) -> (7.7694, 49.5941) centre (0, 49.3) ccw
  line L4 (7.7694, 49.0059) -> (7.4404, 44.3)
  constraints: 10 end point, 2 point on circle, 1 centre point
extrude "Extrusion32" cut sketch "Sketch_59" against normal blind 5.6
sketch "Sketch_60" plane through (0, 0, -64.3) normal (0, 0, 1) x (1, 0, 0)
  line L0 (-10.79, 54.3) -> (-10.79, 44.3)
  line L1 (-10.79, 44.3) -> (-7.4404, 44.3)
  line L2 (-7.4404, 44.3) -> (-7.7694, 49.0059)
  arc A0 (-7.7694, 49.5941) -> (-7.7694, 49.0059) centre (0, 49.3) ccw
  line L3 (-7.7694, 49.5941) -> (-7.4404, 54.3)
  line L4 (-7.4404, 54.3) -> (-10.79, 54.3)
  constraints: 10 end point, 2 point on circle, 1 centre point
extrude "Extrusion33" cut sketch "Sketch_60" against normal blind 5.6
ref_plane "ANBAU_XY" through (0, 0, 0) normal (0, 0, -1) x (1, 0, 0)
ref_plane "ANBAU_YZ" through (0, 0, 0) normal (1, 0, 0) x (0, -1, 0)
ref_plane "ANBAU_ZX" through (0, 0, 0) normal (0, -1, 0) x (0, 0, -1)
ref_plane "SCREWS_1_XY" through (-23.57, -23.57, -5) normal (0, 0, 1) x (1, 0, 0)
ref_plane "SCREWS_1_YZ" through (-23.57, -23.57, -5) normal (1, 0, 0) x (0, 1, 0)
ref_plane "SCREWS_1_ZX" through (-23.57, -23.57, -5) normal (0, 1, 0) x (0, 0, 1)
ref_plane "SCREWS_2_XY" through (-23.57, 23.57, -5) normal (0, 0, 1) x (1, 0, 0)
ref_plane "SCREWS_2_YZ" through (-23.57, 23.57, -5) normal (1, 0, 0) x (0, 1, 0)
ref_plane "SCREWS_2_ZX" through (-23.57, 23.57, -5) normal (0, 1, 0) x (0, 0, 1)
ref_plane "SCREWS_3_XY" through (23.57, -23.57, -5) normal (0, 0, 1) x (1, 0, 0)
ref_plane "SCREWS_3_YZ" through (23.57, -23.57, -5) normal (1, 0, 0) x (0, 1, 0)
ref_plane "SCREWS_3_ZX" through (23.57, -23.57, -5) normal (0, 1, 0) x (0, 0, 1)
ref_plane "SCREWS_4_XY" through (23.57, 23.57, -5) normal (0, 0, 1) x (1, 0, 0)
ref_plane "SCREWS_4_YZ" through (23.57, 23.57, -5) normal (1, 0, 0) x (0, 1, 0)
ref_plane "SCREWS_4_ZX" through (23.57, 23.57, -5) normal (0, 1, 0) x (0, 0, 1)
ref_plane "TO_KABEL_XY" through (0, 49.3, -68.54) normal (0, 0, -1) x (1, 0, 0)
ref_plane "TO_KABEL_YZ" through (0, 49.3, -68.54) normal (1, 0, 0) x (0, -1, 0)
ref_plane "TO_KABEL_ZX" through (0, 49.3, -68.54) normal (0, -1, 0) x (0, 0, -1)
body "Solid1"
